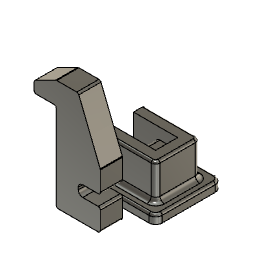
ac_filler_support (Autodesk Fusion 360 design; units mm, degrees)
Autodesk Fusion 360 part; units mm, degrees
sketch "Sketch1" plane through (0, 0, 0) normal (0, 1, 0) x (1, 0, 0)
  line L0 (25, 0) -> (15, 0)
  line L1 (15, 0) -> (15, -40)
  line L2 (25, -15) -> (25, -10)
  line L3 (15, -40) -> (5, -40)
  line L4 (5, -40) -> (5, -45)
  line L5 (15, -50) -> (25, -50)
  line L6 (5, -45) -> (15, -50)
  line L7 (25, 0) -> (35, 0)
  line L8 (35, 0) -> (35, -10)
  line L9 (35, -10) -> (25, -10)
  line L10 (25, -15) -> (35, -15)
  line L11 (35, -15) -> (35, -25)
  line L12 (35, -25) -> (25, -50)
  constraint horizontal L0
  constraint vertical L1
  constraint vertical L2
  constraint horizontal L3
  constraint vertical L4
  constraint horizontal L5
  constraint horizontal L7
  constraint vertical L8
  constraint horizontal L9
  constraint perpendicular L2 L10
  constraint perpendicular L10 L11
extrude "Extrude1" add sketch "Sketch1" along normal blind 10 makes body 1
fillet "Fillet1" radius 1 10 edges at (15, 5, 50) (25, 5, 50) (35, 5, 25) (5, 5, 45) (5, 5, 40) (15, 5, 40) (15, 5, 0) (35, 5, 0) (35, 5, 10) (35, 5, 15) on bodies 1
fillet "Fillet2" radius 2 2 edges at (25, 5, 15) (25, 5, 10) on bodies 1
sketch "Sketch7" plane through (0, 0, 0) normal (0, 0, 1) x (1, 0, 0)
  line L0 (45, 15) -> (15, 15)
  line L1 (15, 45) -> (45, 45)
  line L2 (45, 45) -> (45, 15)
  line L3 (15, 35) -> (35, 35)
  line L4 (35, 35) -> (35, 25)
  line L5 (35, 25) -> (15, 25)
  line L6 (15, 15) -> (15, 25)
  line L7 (15, 35) -> (15, 45)
  constraint horizontal L0
  constraint vertical L6
  constraint horizontal L1
  constraint vertical L2
  constraint horizontal L3
  constraint vertical L4
  constraint horizontal L5
  constraint coincident L3.start L6
  constraint collinear L6 L7
extrude "Extrude7" add sketch "Sketch7" along normal blind 4 separate body makes body 2
sketch "Sketch8" plane through (0, 0, 4) normal (0, 0, 1) x (-1, 0, 0)
  line L0 (-35, -35) -> (-35, -25)
  line L1 (-35, -25) -> (-15, -25)
  line L2 (-15, -25) -> (-15, -15)
  line L3 (-15, -15) -> (-45, -15)
  line L4 (-45, -15) -> (-45, -45)
  line L5 (-45, -45) -> (-15, -45)
  line L6 (-15, -45) -> (-15, -35)
  line L7 (-15, -35) -> (-35, -35)
  line L8 (-15, -40) -> (-40, -40)
  line L9 (-40, -40) -> (-40, -20)
  line L10 (-40, -20) -> (-15, -20)
  line L11 (-15, -25) -> (-35, -25)
  line L12 (-35, -35) -> (-15, -35)
  constraint midpoint L6 L8.start
  constraint perpendicular L6 L8
  constraint perpendicular L8 L9
  constraint midpoint L2 L10.end
  constraint perpendicular L2 L10
  constraint coincident L1.end L2.start
  constraint coincident L0.end L1.start
  constraint coincident L0.start L7.end
  constraint coincident L6.end L7.start
extrude "Extrude8" add sketch "Sketch8" along normal blind 6 contours L0 L1 L2 L6 L7 L8 L9 L10 L11 L12 bodies 2
sketch "Sketch10" plane through (0, 0, 10) normal (0, 0, 1) x (-1, 0, 0)
  line L0 (-15, -25) -> (-15, -20)
  line L1 (-15, -20) -> (-40, -20)
  line L2 (-40, -20) -> (-40, -40)
  line L3 (-40, -40) -> (-15, -40)
  line L4 (-15, -40) -> (-15, -35)
  line L5 (-15, -35) -> (-35, -35)
  line L6 (-35, -35) -> (-35, -25)
  line L7 (-35, -25) -> (-15, -25)
  line L8 (-15, -40) -> (-40, -40)
  line L9 (-40, -20) -> (-15, -20)
  line L10 (-15, -25) -> (-25, -25)
  line L11 (-25, -35) -> (-15, -35)
  line L12 (-25, -35) -> (-25, -25)
  constraint coincident L3.end L4.start
  constraint coincident L2.end L3.start
  constraint coincident L1.end L2.start
  constraint coincident L0.end L1.start
  constraint coincident L0.start L7.end
  constraint midpoint L7 L10.end
  constraint midpoint L5 L11.start
  constraint coincident L4.end L5.start
extrude "Extrude9" add sketch "Sketch10" along normal blind 5 bodies 2
sketch "Sketch11" plane through (0, 0, 15) normal (0, 0, 1) x (-1, 0, 0)
  line L0 (-15, -40) -> (-15, -35)
  line L1 (-15, -35) -> (-25, -35)
  line L2 (-25, -35) -> (-25, -25)
  line L3 (-25, -25) -> (-15, -25)
  line L4 (-15, -25) -> (-15, -20)
  line L5 (-15, -20) -> (-40, -20)
  line L6 (-40, -20) -> (-40, -40)
  line L7 (-40, -40) -> (-15, -40)
  line L8 (-15, -40) -> (-40, -40)
  line L9 (-40, -20) -> (-15, -20)
  line L10 (-15, -25) -> (-35, -25)
  line L11 (-35, -25) -> (-35, -35)
  line L12 (-35, -35) -> (-15, -35)
  constraint coincident L0.start L7.end
  constraint coincident L6.end L7.start
  constraint coincident L5.end L6.start
  constraint coincident L4.end L5.start
  constraint coincident L3.end L4.start
  constraint perpendicular L2 L10
  constraint perpendicular L3 L11
  constraint coincident L0.end L1.start
  constraint perpendicular L0 L12
extrude "Extrude10" add sketch "Sketch11" along normal blind 5 contours L0 L1 L3 L4 L5 L6 L7 L8 L9 L10 L11 L12 bodies 2
fillet "Fillet11" radius 3 2 edges at (45, 15, 2) (45, 45, 2) on bodies 2
fillet "Fillet12" radius 2 2 edges at (40, 20, 12) (40, 40, 12) on bodies 2
fillet "Fillet13" radius 1 10 edges at (28.5, 15, 4) (44.1213, 15.8787, 4) (45, 30, 4) (44.1213, 44.1213, 4) (28.5, 45, 4) (26.5, 20, 20) (39.4142, 20.5858, 20) (40, 30, 20) (39.4142, 39.4142, 20) (26.5, 40, 20) on bodies 2
fillet "Fillet14" radius 2 5 edges at (26.5, 40, 4) (39.4142, 39.4142, 4) (40, 30, 4) (39.4142, 20.5858, 4) (26.5, 20, 4) on bodies 2
fillet "Fillet15" radius 1 1 edges at (35, 30, 15) on bodies 2
fillet "Fillet16" radius 2 2 edges at (25, 30, 15) (25, 30, 10) on bodies 2
